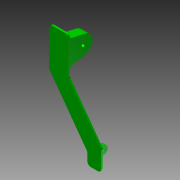
# Autodesk Inventor part: TableMount-Holder
Saved by Autodesk Inventor 2012 (Build 160160000, 160)
## iProperties
Created: 2013-07-16
Part Number: TableMount-Holder
Material: ABS Plastic
Document SubType Name: Modeling
Designer: joe_000
Density: 1.06 g/cm^3
Mass: 86.3684 g
Surface Area: 514.568 cm^2
Volume: 81.4797 cm^3
Author: joe_000
Autodesk Inventor part; units mm, degrees
ref_plane "YZ Plane" through (0, 0, 0) normal (1, 0, 0) x (0, 1, 0)
ref_plane "XZ Plane" through (0, 0, 0) normal (0, 1, 0) x (-1, 0, 0)
sketch "Sketch1" plane through (0, 0, 0) normal (0, 0, 1) x (1, 0, 0)
  line L0 (0, 0) -> (120, 0)
  line L1 (120, 0) -> (120, 198.5)
  line L2 (120, 198.5) -> (0, 198.5)
  line L3 (0, 198.5) -> (0, 0)
  dimension "d0" = 120
  dimension "d1" = 198.5
  constraints: 8 end point, 2 parallel, 1 horizontal, 1 perpendicular
  measures "d0" distance of L1.end L2.end
  measures "d1" distance of L0.end L1.end
extrude "Extrusion1" add sketch "Sketch1" along normal blind 1.5875
ref_plane "Work Plane1" through (60, 0, 0) normal (1, 0, 0) x (0, 0, -1)
sketch "Sketch2" plane through (60, 0, 0) normal (1, 0, 0) x (0, 0, -1)
  line L0 (0, 161.8288) -> (19.05, 157.6055)
  line L1 (0, 136.4288) -> (19.05, 140.6521)
  line L2 (0, 178.6416) -> (0, 113.5366)
  arc A0 (19.05, 140.6521) -> (19.05, 157.6055) centre (17.1708, 149.1288) ccw
  circle A1 centre (17.1708, 149.1288) radius 1.5
  line L3 (0, 0) -> (0, 198.5) projected
  dimension "d4" = 25.4
  dimension "d7" = 19.05
  dimension "d8" = 102.5
  dimension "d9" = 102.5
  dimension "d10" = 3
  constraints: 6 end point, 3 point on line, 2 centre point, 2 point on circle, 1 coincident, 1 tangent, 1 vertical, 1 vertical alignment
  measures "d4" distance of L1.start L0.start
  measures "d7" horizontal distance of L1.start L1.end
  measures "d8" angle of L3 L0
  measures "d9" angle of L3 L1
  measures "d10" diameter of A1
extrude "Extrusion2" add sketch "Sketch2" along normal mid plane 8.0433
fillet "Fillet1" radius 3.175 2 edges at (60, 136.4288, 0) (60, 161.8288, 0)
ref_plane "Work Plane2" through (93.02, 0, 0) normal (1, 0, 0) x (0, 0, -1)
sketch "Sketch3" plane through (93.02, 0, 0) normal (1, 0, 0) x (0, 0, -1)
  line L0 (0, 90.7562) -> (6.35, 89.3485)
  line L1 (0, 80.5013) -> (6.35, 81.9091)
  line L2 (0, 0) -> (0, 198.5) projected
  arc A0 (6.35, 81.9091) -> (6.35, 89.3485) centre (5.5254, 85.6288) ccw
  circle A1 centre (5.5254, 85.6288) radius 0.635
  circle A2 centre (17.1708, 149.1288) radius 1.5 projected
  line L3 (0, 90.7562) -> (0, 80.5013)
  dimension "d14" = 6.35
  dimension "d15" = 102.5
  dimension "d16" = 102.5
  dimension "d17" = 1.27
  dimension "d18" = 3.175
  dimension "d19" = 63.5
  constraints: 6 end point, 2 centre point, 2 point on circle, 2 vertical alignment, 1 coincident, 1 collinear, 1 point on line, 1 tangent
  measures "d14" horizontal distance of L0.start L0.end
  measures "d15" angle of L2 L0
  measures "d16" angle of L2 L1
  measures "d17" diameter of A1
  measures "d18" radial gap between concentric circles of A0 A1
  measures "d19" vertical distance of A2.centre A1.centre
extrude "Extrusion3" add sketch "Sketch3" along normal mid plane 3.175 contours L0 A0 L1 L2
fillet "Fillet2" radius 3.175 2 edges at (93.02, 90.7562, 0) (93.02, 80.5013, 0)
sketch "Sketch6" plane through (0, 0, 0) normal (0, 0, -1) x (-1, 0, 0)
  line L0 (0, 0) -> (-120, 0) projected
  line L1 (0, 198.5) -> (0, 0) projected
  line L2 (-120, 198.5) -> (0, 198.5) projected
  line L3 (-120, 0) -> (-120, 198.5) projected
  line L4 (-89.7815, 73.1271) -> (-96.2585, 73.1271)
  line L5 (-65.7573, 169.203) -> (-54.3273, 169.203)
  line L6 (-51.1523, 166.028) -> (-51.1523, 133.8806)
  line L7 (-51.7557, 132.0185) -> (-86.0031, 84.7203)
  line L8 (-86.6065, 82.8583) -> (-86.6065, 76.3021)
  arc A0 (-86.0031, 84.7203) -> (-86.6065, 82.8583) centre (-83.4315, 82.8583) ccw
  arc A1 (-51.1523, 166.028) -> (-54.3273, 169.203) centre (-54.3273, 166.028) ccw
  arc A2 (-51.7557, 132.0185) -> (-51.1523, 133.8806) centre (-54.3273, 133.8806) ccw
  arc A3 (-89.7815, 73.1271) -> (-86.6065, 76.3021) centre (-89.7815, 76.3021) ccw
  arc A4 (-99.4335, 76.3021) -> (-96.2585, 73.1271) centre (-96.2585, 76.3021) ccw
  line L9 (-55.9783, 164.377) -> (-64.0217, 164.377) projected
  line L10 (-99.4335, 76.3021) -> (-99.4335, 91.129)
  line L11 (-98.8301, 92.991) -> (-69.5357, 133.4487)
  line L12 (-68.9323, 135.3108) -> (-68.9323, 166.028)
  arc A5 (-65.7573, 169.203) -> (-68.9323, 166.028) centre (-65.7573, 166.028) ccw
  arc A6 (-98.8301, 92.991) -> (-99.4335, 91.129) centre (-96.2585, 91.129) ccw
  arc A7 (-69.5357, 133.4487) -> (-68.9323, 135.3108) centre (-72.1073, 135.3108) ccw
  line L13 (-55.9783, 164.377) -> (-55.9783, 133.8806) projected
  line L14 (-64.0217, 133.8806) -> (-64.0217, 164.377) projected
  line L15 (-94.6075, 77.9531) -> (-94.6075, 93.3044) projected
  line L16 (-91.4325, 93.3044) -> (-91.4325, 77.9531) projected
  line L17 (-94.6075, 77.9531) -> (-91.4325, 77.9531) projected
  line L18 (-64.0217, 133.8806) -> (-55.9783, 133.8806) projected
  dimension "d24" = 3.175
  dimension "d27" = 3.175
  dimension "d28" = 15.24
  dimension "d30" = 17.78
  dimension "d31" = 3.175
  dimension "d32" = 3.175
  dimension "d33" = 3.175
  dimension "d34" = 3.175
  dimension "d35" = 3.175
  dimension "d36" = 3.175
  dimension "d37" = 4.826
  dimension "d38" = 4.9107
  dimension "d39" = 4.826
  dimension "d40" = 4.826
  dimension "d41" = 4.826
  dimension "d43" = 4.826
  constraints: 16 end point, 16 point on circle, 16 tangent, 8 centre point, 4 equal radius, 3 parallel, 2 perpendicular, 1 point on line
  measures "d24" radius of A0
  measures "d27" radius of A5
  measures "d28" distance between parallel lines of L7 L11
  measures "d30" distance between parallel lines of L6 L12
  measures "d31" radius of A1
  measures "d32" radius of A7
  measures "d33" radius of A2
  measures "d34" radius of A6
  measures "d35" radius of A4
  measures "d36" radius of A3
  measures "d37" distance between parallel lines of L6 L13
  measures "d38" distance between parallel lines of L12 L14
  measures "d39" distance between parallel lines of L5 L9
  measures "d40" distance between parallel lines of L16 L8
  measures "d41" distance between parallel lines of L4 L17
  measures "d43" distance between parallel lines of L10 L15
extrude "Extrusion4" cut sketch "Sketch6" against normal through all contours L0 L3 L2 L1
equation "\"d0\" = TabletWidth"
equation "\"d1\" = TabletHeight"
equation "\"d4\" = PivotWidth"
equation "\"d7\" = PivotHeight"
equation "\"d8\" = PivotAngle"
equation "\"d9\" = PivotAngle"
equation "\"d10\" = HingeHoleDiameter"
equation "\"d22\" = d18"
equation "\"d15\" = PivotAngle"
equation "\"d16\" = PivotAngle"
equation "\"d20\" = d18"
equation "\"d23\" = d18"
equation "\"d24\" = d18"
equation "\"d27\" = d18"
equation "\"d31\" = d18"
equation "\"d39\" = d37"
equation "\"d40\" = d37"
equation "\"d41\" = d37"
equation "\"d43\" = d37"
equation "\"TabletWidth\" = 120"
equation "\"TabletHeight\" = 198.5"
equation "\"PivotWidth\" = 25.4"
equation "\"PivotHeight\" = 19.05"
equation "\"PivotAngle\" = 102.5deg"
equation "\"HingeHoleDiameter\" = 3"
body "Solid1"
